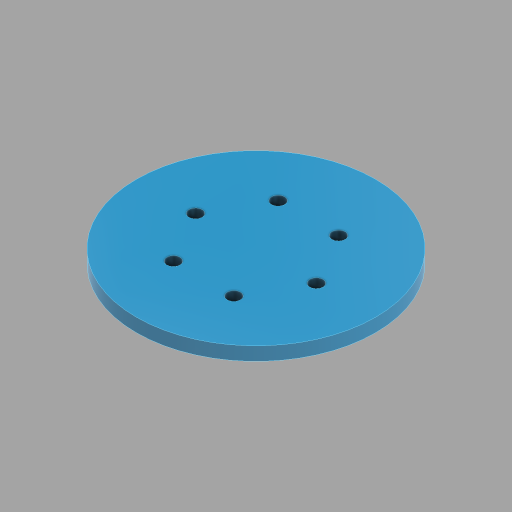
# Autodesk Inventor part: EpoxyFitThroughKF16_mask
Saved by Autodesk Inventor 2024 (Build 280153020, 153B)
## iProperties
Created: 2023-10-02
Part Number: EpoxyFitThroughKF16_mask
Material: Epoxy Resin
Document SubType Name: Modeling
Designer: schanen
Density: 1.14 g/cm^3
Appearance: Sky Blue Dark
Author: schanen
Autodesk Inventor part; units mm, degrees
ref_plane "YZ Plane" through (0, 0, 0) normal (1, 0, 0) x (0, 1, 0)
ref_plane "XZ Plane" through (0, 0, 0) normal (0, 1, 0) x (-1, 0, 0)
ref_plane "XY Plane" through (0, 0, 0) normal (0, 0, 1) x (1, 0, 0)
sketch "Sketch1" plane through (0, 0, 0) normal (0, 1, 0) x (-1, 0, 0)
  circle A0 centre (0, 0) radius 8.9
  dimension "d0" = 17.8
  constraints: 1 centre point, 1 coincident
  measures "d0" diameter of A0
extrude "Extrusion1" add sketch "Sketch1" along normal blind 1
sketch "Sketch2" plane through (0, 1, 0) normal (0, 1, 0) x (1, 0, 0)
  point P0 (0, 0)
  point P1 (-4.5, 0)
  dimension "d4" = 4.5
  measures "d4" distance of point (0, 0) point (-4.5, 0)
hole "Hole1" at (-4.5, 1, 0) direction (0, -1, 0) diameter 1 end through all
pattern_circular "Circular Pattern1" count 6 over 360 about axis through (0, 0, 0) along (0, 1, 0) of "Hole1"
body "Solid1"
